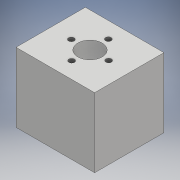
# Autodesk Inventor part: SuporteCastanhaTr8
Saved by Autodesk Inventor 2018 (Build 220112000, 112)
## iProperties
Created: 2018-09-20
Part Number: SuporteCastanhaTr8
Material: Genérico
Document SubType Name: Modeling
Designer: Georgines
Density: 1 g/cm^3
Appearance: Padrão
Author: Georgines
Autodesk Inventor part; units mm, degrees
ref_plane "YZ Plane" through (0, 0, 0) normal (1, 0, 0) x (0, 1, 0)
ref_plane "XZ Plane" through (0, 0, 0) normal (0, 1, 0) x (-1, 0, 0)
ref_plane "XY Plane" through (0, 0, 0) normal (0, 0, 1) x (1, 0, 0)
sketch "Esboço1" plane through (0, 0, 0) normal (0, 0, 1) x (1, 0, 0)
  line L0 (-17, 15) -> (17, 15)
  line L1 (17, 15) -> (17, -15)
  line L2 (17, -15) -> (-17, -15)
  line L3 (-17, -15) -> (-17, 15)
  line L4 (-17, 15) -> (17, -15) construction
  line L5 (17, 15) -> (-17, -15) construction
  point P0 (0, 0)
  dimension "d0" = 34
  dimension "d1" = 30
  constraints: 12 end point, 2 midpoint, 2 parallel, 1 horizontal, 1 perpendicular
  measures "d0" distance of L1.end L2.end
  measures "d1" distance of L0.end L1.end
extrude "Extrusão1" add sketch "Esboço1" along normal blind 30
sketch "Esboço2" plane through (0, 0, 30) normal (0, 0, 1) x (1, 0, 0)
  circle A0 centre (0, 0) radius 8 construction
  circle A1 centre (-0.0751, 7.9996) radius 1 construction
  circle A2 centre (0, 0) radius 8 construction
  circle A3 centre (-7.9996, -0.0751) radius 1 construction
  circle A4 centre (0, 0) radius 8 construction
  circle A5 centre (0.0751, -7.9996) radius 1 construction
  circle A6 centre (0, 0) radius 8 construction
  circle A7 centre (7.9996, 0.0751) radius 1 construction
  dimension "d4" = 16
  dimension "d5" = 2
  dimension "d8" = 360
  constraints: 4 centre point, 3 coincident, 27 other
  measures "d5" diameter of A1
hole "Furo1" at (-0.0751, 7.9996, 30) at (-7.9996, -0.0751, 30) at (7.9996, 0.0751, 30) at (0.0751, -7.9996, 30) direction (0, 0, -1) diameter 2.459 depth 8 tip angle 118 thread size "M3x0.5" class "6H" standard "ANSI Metric M Profile"
sketch "Esboço3" plane through (0, 0, 30) normal (0, 0, 1) x (1, 0, 0)
  circle A0 centre (0, 0) radius 5.25
  dimension "d17" = 10.5
  constraints: 1 centre point, 1 coincident
  measures "d17" diameter of A0
hole "Furo2" at (0, 0, 30) direction (0, 0, -1) diameter 10.5 end through all
sketch "Esboço4" plane through (-17, 15, 0) normal (0, 1, 0) x (1, 0, 0)
  line L0 (0, 0) -> (0, -30) construction
  line L1 (0, -15) -> (34, -15) construction
  line L2 (34, 0) -> (34, -30) construction
  line L3 (18.1544, -30) -> (15.6954, -30) construction
  line L4 (16.9249, -30) -> (17, 0) construction
  line L5 (11.75, 0) -> (22.25, 0) construction
  circle A0 centre (4.9874, -5) radius 1 construction
  circle A1 centre (28.9875, -5) radius 1 construction
  circle A2 centre (28.9374, -25) radius 1 construction
  circle A3 centre (4.9374, -25) radius 1 construction
  dimension "d25" = 2
  dimension "d26" = 2
  dimension "d27" = 2
  dimension "d28" = 2
  dimension "d29" = 10
  dimension "d30" = 10
  dimension "d31" = 10
  dimension "d32" = 10
  dimension "d33" = 12
  dimension "d34" = 12
  dimension "d35" = 12
  dimension "d36" = 12
  constraints: 4 centre point, 4 end point, 4 midpoint
  measures "d25" diameter of A0
  measures "d26" diameter of A1
  measures "d27" diameter of A2
  measures "d28" diameter of A3
  measures "d29" distance from line of L1 A0.centre
  measures "d30" distance from line of L1 A3.centre
  measures "d31" distance from line of L1 A2.centre
  measures "d32" distance from line of L1 A1.centre
  measures "d33" distance from line of L4 A1.centre
  measures "d34" distance from line of L4 A0.centre
  measures "d35" distance from line of L4 A3.centre
  measures "d36" distance from line of L4 A2.centre
hole "Furo3" at (-12.0626, 15, 25) at (-12.0126, 15, 5) at (11.9875, 15, 5) at (11.9374, 15, 25) direction (0, -1, 0) diameter 3.242 depth 12 tip angle 118 thread size "M4x0.7" class "6H" standard "ANSI Metric M Profile"
equation "\"d30\" = d29"
equation "\"d31\" = d29"
equation "\"d32\" = d29"
equation "\"d34\" = d33"
equation "\"d35\" = d33"
equation "\"d36\" = d33"
